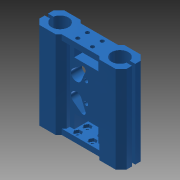
# Autodesk Inventor part: ChimeraXCarriage3
Saved by Autodesk Inventor 2015 SP1 (Build 190203100, 203)
## iProperties
Created: 2014-12-05
Part Number: ChimeraXCarriage3
Material: Generic
Document SubType Name: Modeling
Designer: Jack
Density: 1 g/cm^3
Appearance: Cyan
Author: Jack
Autodesk Inventor part; units mm, degrees
ref_plane "YZ Plane" through (0, 0, 0) normal (1, 0, 0) x (0, 1, 0)
ref_plane "XZ Plane" through (0, 0, 0) normal (0, 1, 0) x (-1, 0, 0)
ref_plane "XY Plane" through (0, 0, 0) normal (0, 0, 1) x (1, 0, 0)
sketch "Sketch1" plane through (0, 0, 0) normal (0, 0, 1) x (1, 0, 0)
  arc A0 (-7.6035, -1.5) -> (-7.6035, 1.5) centre (0, 0) ccw
  arc A1 (62.6035, 1.5) -> (62.6035, -1.5) centre (55, 0) ccw
  line L0 (-12.5, 11.5) -> (67.5, 11.5)
  line L1 (67.5, -11.5) -> (-12.5, -11.5)
  line L2 (-12.5, 1.5) -> (-7.6035, 1.5)
  line L3 (-12.5, -1.5) -> (-7.6035, -1.5)
  line L4 (-12.5, -11.5) -> (-12.5, -1.5)
  line L5 (-12.5, 1.5) -> (-12.5, 11.5)
  line L6 (67.5, 1.5) -> (62.6035, 1.5)
  line L7 (67.5, -1.5) -> (62.6035, -1.5)
  line L8 (67.5, 11.5) -> (67.5, 1.5)
  line L9 (67.5, -1.5) -> (67.5, -11.5)
  dimension "d0" = 15.5
  dimension "d1" = 15.5
  dimension "d2" = 55
  dimension "d3" = 11.5
  dimension "d4" = 11.5
  dimension "d7" = 1.5
  dimension "d8" = 3
  dimension "d9" = 12.5
  dimension "d10" = 12.5
  constraints: 20 end point, 6 perpendicular, 4 point on circle, 3 horizontal, 3 horizontal alignment, 2 centre point, 2 vertical, 2 vertical alignment, 1 coincident, 1 parallel
  measures "d0" diameter of A0
  measures "d1" diameter of A1
  measures "d2" distance of point (0, 0) A1.centre
  measures "d3" distance from line of point (0, 0) L1
  measures "d4" distance from line of L0 point (0, 0)
  measures "d7" distance from line of A1.centre L7
  measures "d8" distance between parallel lines of L6 L7
  measures "d9" distance from line of point (0, 0) L5
  measures "d10" distance from line of L8 A1.centre
extrude "Extrusion1" add sketch "Sketch1" along normal blind 80
chamfer "Chamfer1" distance 5 angle 45 4 edges at (-12.5, 11.5, 40) (-12.5, -11.5, 40) (67.5, 11.5, 40) (67.5, -11.5, 40)
sketch "Sketch2" plane through (0, 0, 80) normal (0, 0, 1) x (1, 0, 0)
  arc A0 (62.6035, 1.5) -> (62.6035, -1.5) centre (55, 0) ccw projected
  line L0 (62.5, 11.5) -> (-7.5, 11.5) projected
  arc A1 (-7.6035, -1.5) -> (-7.6035, 1.5) centre (0, 0) ccw projected
  line L1 (-7.5, -11.5) -> (62.5, -11.5) projected
  line L2 (-7.5, -11.5) -> (62.5, -11.5) projected
  line L3 (7.5, -11.5) -> (12.5, -6.5)
  line L4 (12.5, -6.5) -> (12.5, -3.5)
  line L5 (12.5, -3.5) -> (42.5, -3.5)
  line L6 (42.5, -3.5) -> (42.5, -6.5)
  line L7 (42.5, -6.5) -> (47.5, -11.5)
  line L8 (7.5, 11.5) -> (12.5, 6.5)
  line L9 (12.5, 6.5) -> (12.5, 6.5)
  line L10 (12.5, 6.5) -> (42.5, 6.5)
  line L11 (42.5, 6.5) -> (42.5, 6.5)
  line L12 (42.5, 6.5) -> (47.5, 11.5)
  dimension "d16" = 135
  dimension "d17" = 12.5
  dimension "d18" = 12.5
  dimension "d19" = 5
  dimension "d64" = 45
  dimension "d65" = 45
  dimension "d66" = 10
  dimension "d67" = 6.5
  constraints: 20 end point, 6 perpendicular, 4 point on line, 2 equal length, 2 vertical alignment, 1 horizontal alignment, 1 vertical
  measures "d16" angle of L1 L7
  measures "d17" distance from line of L4 A1.centre
  measures "d18" distance from line of A0.centre L6
  measures "d19" horizontal distance of L3.start L3.end
  measures "d64" angle of L0 L12
  measures "d65" angle of L0 L8
  measures "d66" distance between parallel lines of L5 L10
  measures "d67" distance from line of A0.centre L10
extrude "Extrusion2" cut sketch "Sketch2" against normal up to next
sketch "Sketch3" plane through (12.5, -3.5, 80) normal (0, -1, 0) x (1, 0, 0)
  line L0 (30, -80) -> (0, -80) projected
  line L1 (0, 0) -> (0, -80) projected
  circle A0 centre (15, -49) radius 1.75
  circle A1 centre (15, -31) radius 1.75
  point P0 (-12.5, -80)
  dimension "d23" = 18
  dimension "d24" = 15
  dimension "d25" = 31
  dimension "d26" = 3.5
  constraints: 2 centre point, 1 equal radius, 1 vertical alignment
  measures "d23" distance of A1.centre A0.centre
  measures "d24" distance from line of L1 A1.centre
  measures "d25" distance from line of L0 A0.centre
  measures "d26" diameter of A0
extrude "Extrusion3" cut sketch "Sketch3" against normal up to next
sketch "Sketch4" plane through (12.5, -3.5, 80) normal (0, -1, 0) x (1, 0, 0)
  circle A0 centre (15, -49) radius 1.75 projected
  circle A1 centre (15, -31) radius 1.75 projected
  circle A2 centre (6, -49) radius 5
  circle A3 centre (6, -31) radius 5
  point P0 (-12.5, -80)
  dimension "d29" = 10
  dimension "d30" = 9
  constraints: 2 centre point, 2 horizontal alignment, 1 equal radius, 1 vertical alignment
  measures "d29" diameter of A2
  measures "d30" distance of A0.centre A2.centre
extrude "Extrusion4" cut sketch "Sketch4" against normal up to next contours A2 | A3
sketch "Sketch11" plane through (12.5, 6.5, 80) normal (0, 1, 0) x (1, 0, 0)
  line L0 (0, 80) -> (30, 80) projected
  line L1 (30, 0) -> (0, 0) projected
  line L2 (2, 77) -> (28, 77)
  line L3 (28, 77) -> (28, 60.2)
  line L4 (28, 60.2) -> (2, 60.2)
  line L5 (2, 60.2) -> (2, 77)
  line L6 (2, 19.8) -> (28, 19.8)
  line L7 (28, 19.8) -> (28, 3)
  line L8 (28, 3) -> (2, 3)
  line L9 (2, 3) -> (2, 19.8)
  line L10 (30, 0) -> (30, 80) projected
  point P0 (-12.5, 80)
  dimension "d68" = 26
  dimension "d69" = 16.8
  dimension "d70" = 3
  dimension "d71" = 3
  dimension "d117" = 2
  constraints: 16 end point, 4 parallel, 2 horizontal, 2 perpendicular, 1 collinear, 1 point on line, 1 vertical alignment
  measures "d68" distance of L3.end L4.end
  measures "d69" distance of L2.end L3.end
  measures "d70" distance between parallel lines of L0 L2
  measures "d71" distance between parallel lines of L1 L8
  measures "d117" distance between parallel lines of L10 L7
extrude "Extrusion11" add sketch "Sketch11" along normal blind 3
sketch "Sketch12" plane through (12.5, 9.5, 80) normal (0, 1, 0) x (1, 0, 0)
  line L0 (28, 77) -> (2, 77) projected
  line L1 (2, 77) -> (2, 60.2) projected
  line L2 (2, 60.2) -> (28, 60.2) projected
  line L3 (28, 60.2) -> (28, 77) projected
  line L4 (28, 19.8) -> (2, 19.8) projected
  line L5 (2, 19.8) -> (2, 3) projected
  line L6 (2, 3) -> (28, 3) projected
  line L7 (28, 3) -> (28, 19.8) projected
  line L8 (26, 75) -> (4, 75)
  line L9 (4, 75) -> (4, 62.2)
  line L10 (4, 62.2) -> (26, 62.2)
  line L11 (26, 62.2) -> (26, 75)
  line L12 (26, 17.8) -> (4, 17.8)
  line L13 (4, 17.8) -> (4, 5)
  line L14 (4, 5) -> (26, 5)
  line L15 (26, 5) -> (26, 17.8)
  point P0 (-12.5, 80)
  dimension "d75" = 2
  constraints: 16 end point, 1 collinear, 6 other
  measures "d75" distance between parallel lines of L7 L15
extrude "Extrusion12" cut sketch "Sketch12" against normal up to next contours L11 L10 L9 L8 | L15 L14 L13 L12
sketch "Sketch13" plane through (12.5, -3.5, 80) normal (0, -1, 0) x (1, 0, 0)
  line L0 (4, -62.2) -> (26, -62.2) projected
  line L1 (26, -17.8) -> (4, -17.8) projected
  arc A0 (14.2998, -24.2803) -> (10.4873, -21.3096) centre (12, -23.3) ccw
  arc A1 (10.4873, -58.6904) -> (14.2998, -55.7197) centre (12, -56.7) ccw
  line L2 (0, 0) -> (0, -80) projected
  circle A2 centre (6, -49) radius 5 projected
  circle A3 centre (6, -31) radius 5 projected
  line L3 (10.4873, -58.6904) -> (2.9746, -52.9808)
  circle A4 centre (6, -49) radius 5 projected
  line L4 (14.2998, -55.7197) -> (10.5995, -47.0393)
  line L5 (2.9746, -27.0192) -> (10.4873, -21.3096)
  line L6 (14.2998, -24.2803) -> (10.5995, -32.9607)
  point P0 (-12.5, -80)
  dimension "d78" = 5
  dimension "d79" = 5.5
  dimension "d80" = 5.5
  dimension "d84" = 12
  constraints: 10 point on circle, 8 end point, 8 tangent, 2 centre point, 1 equal radius, 1 vertical alignment
  measures "d78" diameter of A1
  measures "d79" distance from line of A0.centre L1
  measures "d80" distance from line of L0 A1.centre
  measures "d84" distance from line of L2 A1.centre
extrude "Extrusion13" cut sketch "Sketch13" against normal up to next contours L6 A3 L5 A0 | L3 A2 L4 A1
sketch "Sketch17" plane through (0, 0, 0) normal (0, 0, -1) x (-1, 0, 0)
  arc A0 (-62.6035, -1.5) -> (-62.6035, 1.5) centre (-55, 0) ccw projected
  line L0 (-42.5, -6.5) -> (-42.5, -3.5) projected
  line L1 (-42.5, -3.5) -> (-12.5, -3.5) projected
  line L2 (-12.5, -3.5) -> (-12.5, -6.5) projected
  line L3 (-42.5, -6.5) -> (-47.5, -11.5) projected
  line L4 (-44.7, -8.7) -> (-10.3, -8.7)
  line L5 (-7.5, -11.5) -> (-12.5, -6.5) projected
  dimension "d93" = 8.7
  constraints: 2 end point, 2 point on line, 1 horizontal
  measures "d93" distance from line of A0.centre L4
extrude "Extrusion16" add sketch "Sketch17" against normal blind 5
sketch "Sketch18" plane through (0, 0, 80) normal (0, 0, 1) x (1, 0, 0)
  line L0 (7.5, -11.5) -> (12.5, -6.5) projected
  line L1 (12.5, -6.5) -> (12.5, -3.5) projected
  line L2 (12.5, -3.5) -> (42.5, -3.5) projected
  line L3 (42.5, -3.5) -> (42.5, -6.5) projected
  line L4 (42.5, -6.5) -> (47.5, -11.5) projected
  line L5 (10.3, -8.7) -> (44.7, -8.7) projected
extrude "Extrusion17" add sketch "Sketch18" against normal blind 5
sketch "Sketch19" plane through (0, 0, 80) normal (0, 0, 1) x (1, 0, 0)
  line L0 (47.5, 11.5) -> (42.5, 6.5) projected
  line L1 (42.5, 6.5) -> (12.5, 6.5) projected
  line L2 (12.5, 6.5) -> (7.5, 11.5) projected
  arc A0 (-7.6035, -1.5) -> (-7.6035, 1.5) centre (0, 0) ccw projected
  line L3 (10.3, 8.7) -> (44.7, 8.7)
  point P0 (42.5, 6)
  dimension "d98" = 8.7
  constraints: 2 end point, 2 point on line, 1 horizontal, 1 other
  measures "d98" distance from line of A0.centre L3
extrude "Extrusion18" add sketch "Sketch19" against normal blind 5
sketch "Sketch20" plane through (0, 0, 0) normal (0, 0, -1) x (-1, 0, 0)
  line L0 (-7.5, 11.5) -> (-12.5, 6.5) projected
  line L1 (-12.5, 6.5) -> (-12.5, 6) projected
  line L2 (-12.5, 6.5) -> (-42.5, 6.5) projected
  line L3 (-42.5, 6) -> (-42.5, 6.5) projected
  line L4 (-42.5, 6.5) -> (-47.5, 11.5) projected
  line L5 (-10.3, 8.7) -> (-44.7, 8.7) projected
  constraints: 1 other
extrude "Extrusion19" add sketch "Sketch20" against normal blind 5
sketch "Sketch21" plane through (0, 0, 0) normal (0, 0, -1) x (-1, 0, 0)
  line L0 (12.5, 6.5) -> (12.5, 1.5) projected
  line L1 (-10.3, 8.7) -> (-44.7, 8.7) projected
  line L2 (-44.7, -8.7) -> (-10.3, -8.7) projected
  circle A0 centre (-34.25, 4.45) radius 1.75
  circle A1 centre (-20.75, 4.45) radius 1.75
  circle A2 centre (-34.25, -4.45) radius 1.75
  circle A3 centre (-20.75, -4.45) radius 1.75
  dimension "d103" = 13.5
  dimension "d104" = 3.5
  dimension "d105" = 4.25
  dimension "d106" = 4.25
  dimension "d107" = 33.25
  constraints: 4 centre point, 3 equal radius, 2 horizontal alignment, 2 vertical alignment
  measures "d103" distance of A1.centre A0.centre
  measures "d104" diameter of A1
  measures "d105" distance from line of L2 A3.centre
  measures "d106" distance from line of L1 A1.centre
  measures "d107" distance from line of L0 A1.centre
extrude "Extrusion20" cut sketch "Sketch21" against normal up to surface (5 mm away)
sketch "Sketch22" plane through (0, 0, 80) normal (0, 0, 1) x (1, 0, 0)
  circle A0 centre (20.75, 4.45) radius 1.75 projected
  circle A1 centre (34.25, 4.45) radius 1.75 projected
  circle A2 centre (34.25, -4.45) radius 1.75 projected
  circle A3 centre (20.75, -4.45) radius 1.75 projected
extrude "Extrusion21" cut sketch "Sketch22" against normal up to surface (5 mm away)
sketch "Sketch23" plane through (38.5, 9.5, 75) normal (0, 0, -1) x (-1, 0, 0)
  circle A0 centre (4.25, -13.95) radius 1.75 projected
  circle A1 centre (17.75, -13.95) radius 1.75 projected
  circle A2 centre (4.25, -5.05) radius 1.75 projected
  circle A3 centre (17.75, -5.05) radius 1.75 projected
  line L0 (14.3436, -13.95) -> (16.0468, -11)
  line L1 (16.0468, -11) -> (19.4532, -11)
  line L2 (19.4532, -11) -> (21.1564, -13.95)
  line L3 (21.1564, -13.95) -> (19.4532, -16.9)
  line L4 (19.4532, -16.9) -> (16.0468, -16.9)
  line L5 (16.0468, -16.9) -> (14.3436, -13.95)
  line L6 (7.6564, -13.95) -> (5.9532, -16.9)
  line L7 (5.9532, -16.9) -> (2.5468, -16.9)
  line L8 (2.5468, -16.9) -> (0.8436, -13.95)
  line L9 (0.8436, -13.95) -> (2.5468, -11)
  line L10 (2.5468, -11) -> (5.9532, -11)
  line L11 (5.9532, -11) -> (7.6564, -13.95)
  line L12 (14.3436, -5.05) -> (16.0468, -2.1)
  line L13 (16.0468, -2.1) -> (19.4532, -2.1)
  line L14 (19.4532, -2.1) -> (21.1564, -5.05)
  line L15 (21.1564, -5.05) -> (19.4532, -8)
  line L16 (19.4532, -8) -> (16.0468, -8)
  line L17 (16.0468, -8) -> (14.3436, -5.05)
  line L18 (7.6564, -5.05) -> (5.9532, -8)
  line L19 (5.9532, -8) -> (2.5468, -8)
  line L20 (2.5468, -8) -> (0.8436, -5.05)
  line L21 (0.8436, -5.05) -> (2.5468, -2.1)
  line L22 (2.5468, -2.1) -> (5.9532, -2.1)
  line L23 (5.9532, -2.1) -> (7.6564, -5.05)
  point P0 (38.5, -9.5)
  dimension "d112" = 5.9
  constraints: 48 end point, 4 coincident, 4 horizontal, 3 equal length, 52 other
  measures "d112" distance between parallel lines of L1 L4
extrude "Extrusion22" cut sketch "Sketch23" against normal blind 2.7
sketch "Sketch24" plane through (16.5, 9.5, 5) normal (0, 0, 1) x (1, 0, 0)
  circle A0 centre (17.75, -13.95) radius 1.75 projected
  circle A1 centre (4.25, -13.95) radius 1.75 projected
  circle A2 centre (4.25, -5.05) radius 1.75 projected
  circle A3 centre (17.75, -5.05) radius 1.75 projected
  circle A4 centre (4.25, -13.95) radius 1.75 projected
  line L0 (7.6564, -13.95) -> (5.9532, -11) projected
  line L1 (5.9532, -16.9) -> (7.6564, -13.95) projected
  line L2 (2.5468, -16.9) -> (5.9532, -16.9) projected
  line L3 (0.8436, -13.95) -> (2.5468, -16.9) projected
  line L4 (2.5468, -11) -> (0.8436, -13.95) projected
  line L5 (5.9532, -11) -> (2.5468, -11) projected
  circle A5 centre (4.25, -5.05) radius 1.75 projected
  line L6 (7.6564, -5.05) -> (5.9532, -2.1) projected
  line L7 (5.9532, -8) -> (7.6564, -5.05) projected
  line L8 (2.5468, -8) -> (5.9532, -8) projected
  line L9 (0.8436, -5.05) -> (2.5468, -8) projected
  line L10 (2.5468, -2.1) -> (0.8436, -5.05) projected
  line L11 (5.9532, -2.1) -> (2.5468, -2.1) projected
  circle A6 centre (17.75, -13.95) radius 1.75 projected
  line L12 (14.3436, -13.95) -> (16.0468, -16.9) projected
  line L13 (16.0468, -11) -> (14.3436, -13.95) projected
  line L14 (19.4532, -11) -> (16.0468, -11) projected
  line L15 (21.1564, -13.95) -> (19.4532, -11) projected
  line L16 (19.4532, -16.9) -> (21.1564, -13.95) projected
  line L17 (16.0468, -16.9) -> (19.4532, -16.9) projected
  circle A7 centre (17.75, -5.05) radius 1.75 projected
  line L18 (14.3436, -5.05) -> (16.0468, -8) projected
  line L19 (16.0468, -2.1) -> (14.3436, -5.05) projected
  line L20 (19.4532, -2.1) -> (16.0468, -2.1) projected
  line L21 (21.1564, -5.05) -> (19.4532, -2.1) projected
  line L22 (19.4532, -8) -> (21.1564, -5.05) projected
  line L23 (16.0468, -8) -> (19.4532, -8) projected
  point P0 (-16.5, -9.5)
extrude "Extrusion23" cut sketch "Sketch24" against normal blind 2.7
sketch "Sketch25" plane through (38.5, 9.5, 77.7) normal (0, 0, -1) x (-1, 0, 0)
  circle A0 centre (17.75, -13.95) radius 1.75 projected
  circle A1 centre (17.75, -5.05) radius 1.75 projected
  line L0 (14.3436, -5.05) -> (16.0468, -2.1) projected
  line L1 (16.0468, -8) -> (14.3436, -5.05) projected
  line L2 (19.4532, -8) -> (16.0468, -8) projected
  line L3 (21.1564, -5.05) -> (19.4532, -8) projected
  line L4 (19.4532, -2.1) -> (21.1564, -5.05) projected
  line L5 (16.0468, -2.1) -> (19.4532, -2.1) projected
  circle A2 centre (4.25, -13.95) radius 1.75 projected
  line L6 (7.6564, -13.95) -> (5.9532, -16.9) projected
  line L7 (5.9532, -11) -> (7.6564, -13.95) projected
  line L8 (2.5468, -11) -> (5.9532, -11) projected
  line L9 (0.8436, -13.95) -> (2.5468, -11) projected
  line L10 (2.5468, -16.9) -> (0.8436, -13.95) projected
  line L11 (5.9532, -16.9) -> (2.5468, -16.9) projected
  circle A3 centre (4.25, -5.05) radius 1.75 projected
  line L12 (7.6564, -5.05) -> (5.9532, -8) projected
  line L13 (5.9532, -2.1) -> (7.6564, -5.05) projected
  line L14 (2.5468, -2.1) -> (5.9532, -2.1) projected
  line L15 (0.8436, -5.05) -> (2.5468, -2.1) projected
  line L16 (2.5468, -8) -> (0.8436, -5.05) projected
  line L17 (5.9532, -8) -> (2.5468, -8) projected
  point P0 (38.5, -9.5)
sketch "Sketch26" plane through (38.5, 9.5, 75) normal (0, 0, -1) x (-1, 0, 0)
  line L0 (16.0468, -8) -> (14.3436, -5.05) projected
  line L1 (14.3436, -5.05) -> (16.0468, -2.1) projected
  line L2 (16.0468, -2.1) -> (19.4532, -2.1) projected
  line L3 (19.4532, -2.1) -> (21.1564, -5.05) projected
  line L4 (21.1564, -5.05) -> (19.4532, -8) projected
  line L5 (19.4532, -8) -> (16.0468, -8) projected
  line L6 (16.0468, -16.9) -> (14.3436, -13.95) projected
  line L7 (14.3436, -13.95) -> (16.0468, -11) projected
  line L8 (16.0468, -11) -> (19.4532, -11) projected
  line L9 (19.4532, -11) -> (21.1564, -13.95) projected
  line L10 (21.1564, -13.95) -> (19.4532, -16.9) projected
  line L11 (19.4532, -16.9) -> (16.0468, -16.9) projected
  line L12 (5.9532, -11) -> (7.6564, -13.95) projected
  line L13 (7.6564, -13.95) -> (5.9532, -16.9) projected
  line L14 (5.9532, -16.9) -> (2.5468, -16.9) projected
  line L15 (2.5468, -16.9) -> (0.8436, -13.95) projected
  line L16 (0.8436, -13.95) -> (2.5468, -11) projected
  line L17 (2.5468, -11) -> (5.9532, -11) projected
  line L18 (5.9532, -2.1) -> (7.6564, -5.05) projected
  line L19 (7.6564, -5.05) -> (5.9532, -8) projected
  line L20 (5.9532, -8) -> (2.5468, -8) projected
  line L21 (2.5468, -8) -> (0.8436, -5.05) projected
  line L22 (0.8436, -5.05) -> (2.5468, -2.1) projected
  line L23 (2.5468, -2.1) -> (5.9532, -2.1) projected
  point P0 (38.5, -9.5)
body "Solid1"
